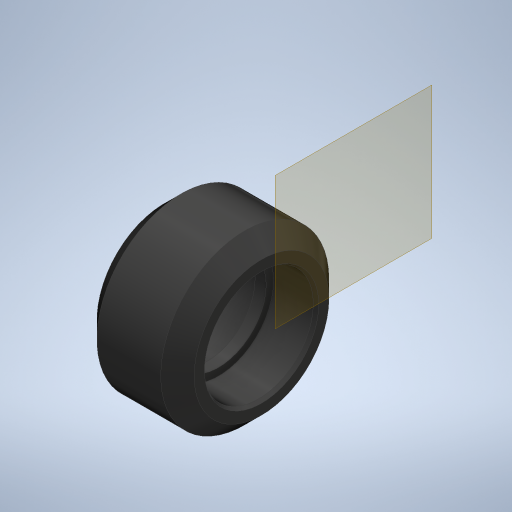
# Autodesk Inventor part: CSW-1523
Saved by Autodesk Inventor 2024.3 (Build 283343000, 343)
## iProperties
Created: 2016-10-14
Part Number: CSW-1523
Material: Типовые
Document SubType Name: Modeling
Designer: skhalipa
Density: 1 g/cm^3
Appearance: Темно-серый
Author: skhalipa
Autodesk Inventor part; units mm, degrees
ref_plane "YZ Plane" through (0, 0, 0) normal (1, 0, 0) x (0, 1, 0)
ref_plane "XY Plane" through (0, 0, 0) normal (0, 0, 1) x (1, 0, 0)
sketch "Эскиз4" plane through (0, 0, 0) normal (0, 0, 1) x (1, 0, 0)
  line L0 (-4.4, 7.615) -> (4.4, 7.615) construction
  line L1 (4.4, 7.615) -> (4.4, -7.615) construction
  line L2 (4.4, -7.615) -> (-4.4, -7.615) construction
  line L3 (-4.4, -7.615) -> (-4.4, 7.615) construction
  line L4 (-2.89, 7.615) -> (-2.89, -7.615) construction
  line L5 (2.89, 7.615) -> (2.89, -7.615) construction
  line L6 (-4.4, 6.105) -> (4.4, 6.105) construction
  line L7 (-4.4, -6.105) -> (4.4, -6.105) construction
  line L8 (-4.4, 5.175) -> (4.4, 5.175) construction
  line L9 (-4.4, -5.175) -> (4.4, -5.175) construction
  line L10 (-4.4, 4.987) -> (4.4, 4.987) construction
  line L11 (-4.4, -4.987) -> (4.4, -4.987) construction
  line L12 (-4.1, 7.615) -> (-4.1, -7.615) construction
  line L13 (4.1, 7.615) -> (4.1, -7.615) construction
  line L14 (-0.5, 7.615) -> (-0.5, -7.615) construction
  line L15 (0.5, 7.615) -> (0.5, -7.615) construction
  line L16 (-4.4, 4.32) -> (4.4, 4.32) construction
  line L17 (-4.4, -4.32) -> (4.4, -4.32) construction
  line L18 (-2.89, 7.615) -> (-4.4, 6.105)
  line L19 (-4.4, 6.105) -> (-4.4, 5.175)
  line L20 (-4.4, 5.175) -> (-4.1, 4.987)
  line L21 (-0.5, 4.987) -> (-4.1, 4.987)
  line L22 (-0.5, 4.32) -> (-0.5, 4.987)
  line L23 (-0.5, 4.32) -> (0.5, 4.32)
  line L24 (0.5, 4.32) -> (0.5, 4.987)
  line L25 (0.5, 4.987) -> (4.1, 4.987)
  line L26 (4.1, 4.987) -> (4.4, 5.175)
  line L27 (4.4, 5.175) -> (4.4, 6.105)
  line L28 (4.4, 6.105) -> (2.89, 7.615)
  line L29 (-2.89, 7.615) -> (2.89, 7.615)
  line L30 (-4.4, 0) -> (4.4, 0)
  point P0 (0, 0)
  point P1 (-4.4, 0)
  point P2 (0, 7.615)
  point P3 (0, 0)
  dimension "d17" = 8.8
  dimension "d18" = 15.23
  dimension "d19" = 5.78
  dimension "d20" = 2.89
  dimension "d21" = 12.21
  dimension "d22" = 6.105
  dimension "d23" = 10.35
  dimension "d24" = 5.175
  dimension "d25" = 9.974
  dimension "d26" = 4.987
  dimension "d27" = 0.3
  dimension "d28" = 0.3
  dimension "d29" = 0.5
  dimension "d30" = 1
  dimension "d31" = 8.64
  dimension "d32" = 4.32
  dimension "d33" = 8.8
  dimension "d34" = 7.615
  constraints: 56 end point, 18 point on line, 11 horizontal, 7 perpendicular, 2 vertical, 1 coincident, 1 collinear, 1 horizontal alignment, 1 midpoint, 1 vertical alignment, 33 other
  measures "d17" distance of point (-4.4, 7.615) point (4.4, 7.615)
  measures "d18" distance of point (4.4, 7.615) L2.start
  measures "d19" distance between parallel lines of L5 L4
  measures "d20" distance from line of point (0, 0) L4
  measures "d21" distance between parallel lines of L7 L6
  measures "d22" distance from line of point (0, 0) L6
  measures "d23" distance between parallel lines of L9 L8
  measures "d24" distance from line of point (0, 0) L8
  measures "d25" distance between parallel lines of L11 L10
  measures "d26" distance from line of point (0, 0) L10
  measures "d29" distance from line of point (0, 0) L14
  measures "d30" distance between parallel lines of L15 L14
  measures "d31" distance between parallel lines of L17 L16
  measures "d32" distance from line of point (0, 0) L16
  measures "d33" distance of L30.end L30.start
  measures "d34" distance of point (0, 0) point (0, 7.615)
revolve "Вращение2" add sketch "Эскиз4" angle 360 about axis through (-4.4, 0, 0) along (1, 0, 0)
ref_plane "РабПлоскость3" through (0, 7.615, 0) normal (0, 1, 0) x (-1, 0, 0)
sketch "Эскиз7" plane through (0, 7.615, 0) normal (0, 1, 0) x (-1, 0, 0)
  point P0 (0, 0)
ref_plane "Work Plane4" through (5.75, 0, 0) normal (1, 0, 0) x (0, 0, -1)
